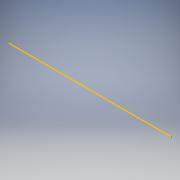
# Autodesk Inventor part: Rail
Saved by Autodesk Inventor 2018.1 (Build 221171000, 171)
## iProperties
Created: 2017-12-03
Part Number: Rail
Material: Generic
Document SubType Name: Modeling
Designer: xdlea
Density: 1 g/cm^3
Appearance: Default(1)
Author: xdlea
Autodesk Inventor part; units mm, degrees
ref_plane "YZ Plane" through (0, 0, 0) normal (1, 0, 0) x (0, 1, 0)
ref_plane "XZ Plane" through (0, 0, 0) normal (0, 1, 0) x (-1, 0, 0)
ref_plane "XY Plane" through (0, 0, 0) normal (0, 0, 1) x (1, 0, 0)
sketch "Sketch1" plane through (0, 0, 0) normal (1, 0, 0) x (0, 1, 0)
  circle A0 centre (0, 0) radius 0.4064
  dimension "d1" = 0.8128
  constraints: 1 centre point, 1 coincident
  measures "d1" diameter of A0
derived "Carriage.ipt"
extrude "Extrusion1" add sketch "Sketch1" along normal mid plane 149.225
equation "\"d1\" = clothesHangerDia"
equation "\"clothesHangerDia\" = 0.8128"
body "Solid1"
